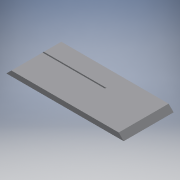
# Autodesk Inventor part: deksel token Edited
Saved by Autodesk Inventor 2018.3 (Build 223284000, 284)
## iProperties
Created: 2020-11-30
Part Number: deksel token Edited
Material: Generic
Document SubType Name: Modeling
Designer: Olivi
Density: 1 g/cm^3
Appearance: Default
Author: Olivi
Autodesk Inventor part; units mm, degrees
ref_plane "YZ Plane" through (0, 0, 0) normal (1, 0, 0) x (0, 1, 0)
ref_plane "XZ Plane" through (0, 0, 0) normal (0, 1, 0) x (-1, 0, 0)
ref_plane "XY Plane" through (0, 0, 0) normal (0, 0, 1) x (1, 0, 0)
sketch "Sketch1" plane through (0, 0, 0) normal (0, 0, 1) x (1, 0, 0)
  line L0 (0, 0) -> (43, 0)
  line L1 (43, 0) -> (43, 20)
  line L2 (43, 20) -> (0, 20)
  line L3 (0, 20) -> (0, 0)
  dimension "d0" = 43
  dimension "d1" = 20
  constraints: 8 end point, 2 parallel, 1 horizontal, 1 perpendicular
  measures "d0" distance of L2.end L1.end
  measures "d1" distance of L1.end L0.end
extrude "Extrusion1" add sketch "Sketch1" along normal blind 2
sketch "Sketch2" plane through (0, 0, 0) normal (0, -1, 0) x (1, 0, 0)
  line L0 (43, 0) -> (43, 2) projected
  line L1 (0, 0) -> (0, 2) projected
  line L2 (0, 0) -> (-2, 0)
  line L3 (-2, 0) -> (0, 2)
  line L4 (43, 0) -> (45, 0)
  line L5 (45, 0) -> (43, 2)
  dimension "d4" = 2
  dimension "d5" = 2
  constraints: 8 end point, 2 horizontal
  measures "d4" distance of L1.start L2.end
  measures "d5" distance of L0.start L4.end
extrude "Extrusion2" add sketch "Sketch2" against normal blind 20
sketch "Sketch5" plane through (0, 0, 2) normal (0, 0, 1) x (1, 0, 0)
  line L0 (0, 0) -> (43, 0) projected
  line L1 (43, 20) -> (0, 20) projected
  line L2 (0, 20) -> (0, 0) projected
  line L3 (5, 5) -> (25, 5)
  line L4 (25, 5) -> (25, 15)
  line L5 (25, 15) -> (5, 15)
  line L6 (5, 15) -> (5, 5)
  dimension "d26" = 20
  dimension "d27" = 10
  dimension "d28" = 5
  dimension "d29" = 5
  dimension "d30" = 5
  constraints: 8 end point, 2 parallel, 1 horizontal, 1 perpendicular
  measures "d26" distance of L5.end L4.end
  measures "d27" distance of L4.end L3.end
  measures "d28" distance between parallel lines of L0 L3
  measures "d29" distance between parallel lines of L1 L5
  measures "d30" distance between parallel lines of L2 L6
extrude "Extrusion5" cut sketch "Sketch5" against normal blind 1.5
sketch "Sketch6" plane through (5, 5, 2) normal (1, 0, 0) x (0, 0, -1)
  line L0 (0, 0) -> (0, 10) projected
  line L1 (0, 0) -> (1.5, 0) projected
  line L2 (1.5, 0) -> (1.5, 10) projected
  line L3 (0, 10) -> (1.5, 10) projected
  point P0 (2, -5)
extrude "Extrusion6" cut sketch "Sketch6" against normal up to next
sketch "Sketch7" plane through (0, 15, 2) normal (0, -1, 0) x (1, 0, 0)
  line L0 (0, 0) -> (25, 0) projected
  line L1 (-1.5, -1.5) -> (0, 0) projected
  line L2 (25, 0) -> (0, 0)
  line L3 (0, 0) -> (0, -0.5)
  line L4 (0, -0.5) -> (25, -0.5)
  line L5 (25, -0.5) -> (25, 0)
  line L6 (0, -0.5) -> (-0.5, -0.5)
  line L7 (0, 0) -> (-0.5, -0.5)
  point P0 (0, -2)
  dimension "d35" = 0.5
  constraints: 12 end point, 2 horizontal, 2 parallel, 1 perpendicular, 1 point on line
  measures "d35" distance of L3.end L2.end
extrude "Extrusion7" add sketch "Sketch7" along normal blind 2
sketch "Sketch8" plane through (0, 5, 2) normal (0, 1, 0) x (1, 0, 0)
  line L0 (0, 0) -> (-1.5, 1.5) projected
  line L1 (25, 0) -> (0, 0)
  line L2 (0, 0) -> (0, 0.5)
  line L3 (0, 0.5) -> (25, 0.5)
  line L4 (25, 0.5) -> (25, 0)
  line L5 (0, 0.5) -> (-0.5, 0.5)
  line L6 (0, 0) -> (-0.5, 0.5)
  point P0 (0, 2)
  dimension "d38" = 25
  dimension "d39" = 0.5
  constraints: 12 end point, 2 horizontal, 2 parallel, 1 perpendicular, 1 point on line
  measures "d38" distance of L2.end L3.end
  measures "d39" distance of L1.end L2.end
extrude "Extrusion8" add sketch "Sketch8" along normal blind 2
body "Solid1"
